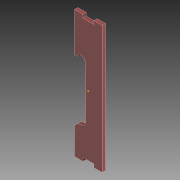
# Autodesk Inventor part: Планка боковая
Saved by Autodesk Inventor 2022 (Build 260153000, 153)
## iProperties
Created: 2025-01-10
Part Number: Планка боковая
Material: Типовые
Document SubType Name: Modeling
Designer: Ivan
Density: 1 g/cm^3
Appearance: Каштановый
Mass: 54.6996 g
Surface Area: 219.565 cm^2
Volume: 54.6996 cm^3
Author: Ivan
Title: Планка боковая
Autodesk Inventor part; units mm, degrees
ref_plane "YZ Plane" through (0, 0, 0) normal (1, 0, 0) x (0, 1, 0)
ref_plane "XZ Plane" through (0, 0, 0) normal (0, 1, 0) x (-1, 0, 0)
ref_plane "XY Plane" through (0, 0, 0) normal (0, 0, 1) x (1, 0, 0)
sketch "Эскиз1" plane through (0, 0, 0) normal (0, 0, 1) x (1, 0, 0)
  line L0 (-25, -109) -> (25, -109)
  line L1 (25, -109) -> (25, 109)
  line L2 (25, 109) -> (-25, 109)
  line L3 (-25, 109) -> (-25, -109)
  line L4 (-25, -109) -> (25, 109) construction
  line L5 (25, -109) -> (-25, 109) construction
  line L6 (0, 0) -> (0, 129.6236) construction
  line L7 (0, 0) -> (116.4638, 0) construction
  line L8 (-25, 109) -> (-10, 109)
  line L9 (-10, 109) -> (-10, 115)
  line L10 (-10, 115) -> (-25, 115)
  line L11 (-25, 115) -> (-25, 109)
  line L12 (25, 109) -> (10, 109)
  line L13 (10, 109) -> (10, 115)
  line L14 (10, 115) -> (25, 115)
  line L15 (25, 115) -> (25, 109)
  line L16 (-25, -109) -> (-10, -109)
  line L17 (-10, -109) -> (-10, -115)
  line L18 (-10, -115) -> (-25, -115)
  line L19 (-25, -115) -> (-25, -109)
  line L20 (25, -109) -> (10, -109)
  line L21 (10, -109) -> (10, -115)
  line L22 (10, -115) -> (25, -115)
  line L23 (25, -115) -> (25, -109)
  dimension "d0" = 50
  dimension "d1" = 15
  dimension "d2" = 6
  dimension "d3" = 230
  constraints: 48 end point, 10 parallel, 6 horizontal, 5 perpendicular, 4 equal length, 2 midpoint, 2 point on line, 1 vertical
  measures "d0" distance of L1.end L2.end
  measures "d1" distance of L13.end L14.end
  measures "d2" distance of L12.end L13.end
  measures "d3" distance between parallel lines of L22 L14
extrude "Выдавливание1" add sketch "Эскиз1" along normal mid plane 6
sketch "Эскиз2" plane through (0, 0, 3) normal (0, 0, 1) x (1, 0, 0)
  point P0 (0, 0)
sketch "Эскиз3" plane through (0, 0, 3) normal (0, 0, 1) x (1, 0, 0)
  line L0 (-41.4458, -60) -> (-5, -60)
  line L1 (-5, -60) -> (-5, 50)
  line L2 (-5, 50) -> (-41.4458, 50)
  line L3 (-41.4458, 50) -> (-41.4458, -60)
  line L4 (-25, -115) -> (-10, -115) projected
  line L5 (-25, 115) -> (-25, -115) projected
  line L6 (-25, 50) -> (-19, 50)
  line L7 (-19, 50) -> (-19, 44)
  line L8 (-19, 44) -> (-25, 44)
  line L9 (-25, 44) -> (-25, 50)
  point P0 (0, 0)
  dimension "d8" = 20
  dimension "d12" = 6
  dimension "d13" = 6
  dimension "d17" = 50
  dimension "d18" = 60
  constraints: 16 end point, 4 perpendicular, 2 horizontal, 2 parallel, 2 point on line
  measures "d8" distance between parallel lines of L5 L1
  measures "d12" distance of L6.end L7.end
  measures "d13" distance of L7.end L8.end
  measures "d17" distance from line of point (0, 0) L2
  measures "d18" distance from line of L0 point (0, 0)
extrude "Выдавливание2" cut sketch "Эскиз3" against normal through all contours L3 L2 L5 L0 | L5 L8 L7 L2 L1 L0
fillet "Сопряжение1" radius 10 3 edges at (-5, -60, 0) (-5, 50, 0) (-25, -60, 0)
fillet "Сопряжение2" radius 2 3 edges at (-19, 44, 0) (-25, 44, 0) (-19, 50, 0)
